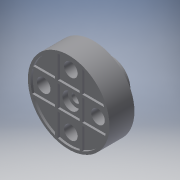
# Autodesk Inventor part: Motor rotor
Saved by Autodesk Inventor 2019 (Build 230136000, 136)
## iProperties
Created: 2018-11-25
Part Number: Motor rotor
Material: Generic
Document SubType Name: Modeling
Designer: Varga Daniel
Density: 1 g/cm^3
Appearance: Default
Mass: 6.08942 g
Surface Area: 33.2818 cm^2
Volume: 6.08942 cm^3
Author: Varga Daniel
Autodesk Inventor part; units mm, degrees
ref_plane "YZ Plane" through (0, 0, 0) normal (1, 0, 0) x (0, 1, 0)
ref_plane "XZ Plane" through (0, 0, 0) normal (0, 1, 0) x (-1, 0, 0)
ref_plane "XY Plane" through (0, 0, 0) normal (0, 0, 1) x (1, 0, 0)
sketch "Sketch1" plane through (0, 0, 0) normal (0, 0, 1) x (1, 0, 0)
  line L0 (0, 0) -> (22.9276, 0) construction
  line L1 (0, 0) -> (0, -25.2472) construction
  circle A0 centre (0, 10) radius 2.5
  circle A1 centre (10, 0) radius 2.5
  circle A2 centre (-10, 0) radius 2.5
  circle A3 centre (0, -10) radius 2.5
  circle A4 centre (0, 0) radius 15
  circle A5 centre (0, 0) radius 1.7
  dimension "d0" = 5
  dimension "d1" = 20
  dimension "d2" = 5
  dimension "d3" = 20
  dimension "d4" = 30
  dimension "d5" = 3.4
  constraints: 6 centre point, 4 end point, 3 coincident, 2 point on line, 2 symmetric about line, 1 horizontal, 1 vertical, 2 other
  measures "d0" diameter of A0
  measures "d1" diameter of A0.centre L0
  measures "d2" diameter of A1
  measures "d3" diameter of A1.centre L1
  measures "d4" diameter of A4
  measures "d5" diameter of A5
extrude "Extrusion1" add sketch "Sketch1" along normal blind 8.4
sketch "Sketch2" plane through (0, 0, 8.4) normal (0, 0, 1) x (1, 0, 0)
  circle A0 centre (0, 0) radius 15 projected
  circle A1 centre (10, 0) radius 2.5 construction
  line L0 (0, 0) -> (10, 0) construction
  line L1 (0, 0) -> (0, -10.0085) construction
  arc A2 (4, 13.4164) -> (-4, 13.4164) centre (0, 0) ccw
  line L2 (-5, 5) -> (-13.0767, 5)
  line L3 (-4, 5) -> (-4, 13.4164)
  line L4 (-5, 5) -> (-5, 13.0767)
  line L5 (-13.4164, 4) -> (-5, 4)
  arc A3 (-5, 13.0767) -> (-13.0767, 5) centre (0, 0) ccw
  arc A4 (-13.4164, 4) -> (-13.4164, -4) centre (0, 0) ccw
  line L6 (-5, -4) -> (-13.4164, -4)
  line L7 (-5, -13.0767) -> (-5, -5)
  line L8 (-5, -4) -> (-5, 4)
  line L9 (-4, -13.4164) -> (-4, -5)
  line L10 (-4, -4) -> (-4, 4)
  line L11 (-5, -5) -> (-13.0767, -5)
  line L12 (4, -13.4164) -> (4, -5)
  line L13 (5, -13.0767) -> (5, -5)
  line L14 (13.0767, -5) -> (5, -5)
  line L15 (4, -5) -> (-4, -5)
  line L16 (13.4164, -4) -> (5, -4)
  line L17 (4, -4) -> (-4, -4)
  line L18 (-4, 4) -> (4, 4)
  line L19 (5, 4) -> (13.4164, 4)
  line L20 (4, -4) -> (4, 4)
  line L21 (4, 5) -> (4, 13.4164)
  line L22 (13.0767, 5) -> (5, 5)
  line L23 (4, 5) -> (-4, 5)
  line L24 (5, -4) -> (5, 4)
  line L25 (5, 5) -> (5, 13.0767)
  arc A5 (13.0767, 5) -> (5, 13.0767) centre (0, 0) ccw
  arc A6 (13.4164, -4) -> (13.4164, 4) centre (0, 0) ccw
  arc A7 (5, -13.0767) -> (13.0767, -5) centre (0, 0) ccw
  arc A8 (-13.0767, -5) -> (-5, -13.0767) centre (0, 0) ccw
  arc A9 (-4, -13.4164) -> (4, -13.4164) centre (0, 0) ccw
  constraints: 52 end point, 18 parallel, 16 point on circle, 8 centre point, 7 horizontal, 7 vertical
extrude "Extrusion2" add sketch "Sketch2" along normal blind 0.8
sketch "Sketch3" plane through (0, 0, 0) normal (0, 0, -1) x (-1, 0, 0)
  line L0 (-1.95, 1.7197) -> (-1.95, -1.7197)
  line L1 (1.95, 1.7197) -> (1.95, -1.7197)
  line L2 (0, 0) -> (0, 3.5197) construction
  arc A0 (1.95, 1.7197) -> (-1.95, 1.7197) centre (0, 0) ccw
  arc A1 (-1.95, -1.7197) -> (1.95, -1.7197) centre (0, 0) ccw
  dimension "d25" = 3.9
  dimension "d26" = 2.6
  dimension "d27" = 2.6
  constraints: 7 end point, 4 point on circle, 2 centre point, 2 vertical, 1 parallel, 1 other
  measures "d25" distance between parallel lines of L0 L1
  measures "d26" radius of A1
  measures "d27" radius of A0
extrude "Extrusion3" cut sketch "Sketch3" against normal blind 2.4
sketch "Sketch4" plane through (0, 0, 0) normal (0, 0, -1) x (-1, 0, 0)
  arc A0 (1.95, 1.7197) -> (-1.95, 1.7197) centre (0, 0) ccw projected
  line L0 (1.95, 1.7197) -> (1.95, -1.7197) projected
  arc A1 (-1.95, -1.7197) -> (1.95, -1.7197) centre (0, 0) ccw projected
  line L1 (-1.95, -1.7197) -> (-1.95, 1.7197) projected
  circle A2 centre (0, 0) radius 7
  dimension "d30" = 14
  constraints: 1 centre point, 1 coincident
  measures "d30" diameter of A2
extrude "Extrusion4" add sketch "Sketch4" along normal blind 6.5
sketch "Sketch7" plane through (0, 0, -6.5) normal (0, 0, -1) x (-1, 0, 0)
  arc A0 (1.95, 1.7197) -> (-1.95, 1.7197) centre (0, 0) ccw construction
  circle A1 centre (0, 0) radius 4
  dimension "d36" = 8
  constraints: 1 centre point, 1 coincident
  measures "d36" diameter of A1
extrude "Extrusion6" cut sketch "Sketch7" against normal blind 0.9
sketch "Sketch5" plane through (0, 0, 8.4) normal (0, 0, 1) x (1, 0, 0)
  circle A0 centre (0, 0) radius 3.1
  dimension "d33" = 6.2
  constraints: 1 centre point, 1 coincident
  measures "d33" diameter of A0
extrude "Extrusion5" cut sketch "Sketch5" against normal blind 2.6
sketch "Sketch6" plane through (0, 0, -6.5) normal (0, 0, -1) x (-1, 0, 0)
  point P0 (0, 0)
chamfer "Chamfer1" distance 1.4 angle 45 4 edges at (1.95, 0, -5.6) (0, -2.6, -5.6) (-1.95, 0, -5.6) (0, 2.6, -5.6)
equation "\"d27\" = d26"
body "Solid1"
